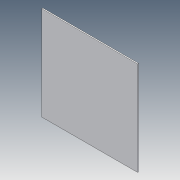
# Autodesk Inventor part: logo
Saved by Autodesk Inventor 2012 (Build 160160000, 160)
## iProperties
Created: 2011-06-06
Part Number: logo
Document SubType Name: Modeling
Designer: dfoster
Density: 1 g/cm^3
Material: Default
Author: dfoster
Autodesk Inventor part; units mm, degrees
ref_plane "YZ Plane" through (0, 0, 0) normal (1, 0, 0) x (0, 1, 0)
ref_plane "XZ Plane" through (0, 0, 0) normal (0, 1, 0) x (-1, 0, 0)
ref_plane "XY Plane" through (0, 0, 0) normal (0, 0, 1) x (1, 0, 0)
sketch "Sketch1" plane through (0, 0, 0) normal (0, 0, 1) x (1, 0, 0)
  line L0 (0, 0) -> (1219.2, 0)
  line L1 (1219.2, 0) -> (1219.2, 1193.8)
  line L2 (1219.2, 1193.8) -> (0, 1193.8)
  line L3 (0, 1193.8) -> (0, 0)
  dimension "d0" = 1193.8
  dimension "d1" = 1219.2
  constraints: 8 end point, 2 parallel, 1 horizontal, 1 perpendicular
  measures "d0" distance between parallel lines of L0 L2
  measures "d1" distance between parallel lines of L1 L3
extrude "Extrusion1" add sketch "Sketch1" along normal blind 12.7
sketch "Sketch2" plane through (0, 0, 0) normal (0, 0, -1) x (-1, 0, 0)
  line L0 (-1219.2, 0) -> (-1219.2, 1193.8) projected
  line L1 (-1689.1, 1117.6) -> (541.6516, 1117.6) construction
  line L2 (541.6516, 1117.6) -> (541.6516, 76.2) construction
  line L3 (541.6516, 76.2) -> (-1689.1, 76.2) construction
  line L4 (-1689.1, 76.2) -> (-1689.1, 1117.6) construction
  line L5 (0, 0) -> (-1219.2, 0) projected
  line L6 (-1219.2, 1193.8) -> (0, 1193.8) projected
  dimension "d24" = 76.2
  dimension "d32" = 76.2
  dimension "d38" = 2230.7516
  dimension "d39" = 469.9
  constraints: 2 other
  measures "d24" distance between parallel lines of L1 L6
  measures "d32" distance between parallel lines of L3 L5
  measures "d38" distance of L2.end L3.end
  measures "d39" distance between parallel lines of L0 L4
decal "Decal1"
body "Solid1"
